Autodesk Fusion 360 part; units mm, degrees
note: some values were not read from the file. Chosen so that the rebuilt part matches the saved one: which bodies a step acts on; which face or edge a step refers to. Set by a fixed rule: which sketch regions a step uses.
(part 2 of 3)
sketch "Sketch1" plane through (0, 0, 0) normal (0, 0, 1) x (1, 0, 0)
  line L0 (10, 10) -> (15, 10)
  line L1 (15, 10) -> (15, 4)
  line L2 (15, 4) -> (10, 4)
  line L3 (10, 4) -> (10, 10)
  line L4 (10, 7) -> (-20, 7) construction
  line L5 (-20, 10) -> (-15, 10)
  line L6 (-15, 10) -> (-15, 4)
  line L7 (-15, 4) -> (-20, 4)
  line L8 (-20, 4) -> (-20, 10)
  dimension "d1" = 5
  dimension "d2" = 6
  dimension "d3" = 30
  dimension "d4" = 5
  dimension "d5" = 6
  constraint horizontal L0
  constraint vertical L1
  constraint horizontal L2
  constraint vertical L3
  constraint midpoint L3 L4.start
  constraint perpendicular L3 L4
  constraint horizontal L5
  constraint vertical L6
  constraint horizontal L7
  constraint vertical L8
  measures "d1" distance of L0.start L0.end
  measures "d2" distance of L0.start L2.end
  measures "d3" distance of L4.start L4.end
  measures "d4" distance of L5.start L5.end
  measures "d5" distance of L5.start L7.end
extrude "Extrude1" add sketch "Sketch1" along normal blind 34.231 makes body 1 at (-15, 8, 11.4103) makes body 2 at (15, 8, 11.4103)
sketch "Sketch2" plane through (-15, 0, 0) normal (1, 0, 0) x (0, 1, 0)
  line L0 (4, 0) -> (10, 0)
  line L1 (10, 0) -> (10, 34.231)
  line L2 (10, 34.231) -> (4, 34.231)
  line L3 (4, 34.231) -> (4, 0)
  line L4 (4, 34.231) -> (10, 34.231)
  line L5 (10, 34.231) -> (10, 29.231)
  line L6 (10, 29.231) -> (4, 29.231)
  line L7 (4, 29.231) -> (4, 34.231)
  dimension "d8" = 5
  constraint horizontal L4
  constraint vertical L5
  constraint horizontal L6
  constraint vertical L7
  constraint coincident L2.end L3.start
  measures "d8" distance of L2.end L6.end
extrude "Extrude2" add sketch "Sketch2" along normal blind 20 contours L1 L2 L3 L4 L5 L6 L7 bodies 1
move_body "Move1" bodies 2 to x (1, 0, 0) y (0, 1, 0) z (0, 0, 1) at (-5, 0, 0)
combine "Combine1" operation add target body 1 tool bodies 2
sketch "Sketch3" plane through (0, 0, 34.231) normal (0, 0, 1) x (-1, 0, 0)
  line L0 (20, -4) -> (-10, -4)
  line L1 (-10, -4) -> (-10, -10)
  line L2 (-10, -10) -> (20, -10)
  line L3 (20, -10) -> (20, -4)
  line L4 (-10, -10) -> (2, -10)
  line L5 (2, -10) -> (2, -4)
  line L6 (2, -4) -> (-10, -4)
  line L7 (-10, -4) -> (-10, -10)
  line L8 (20, -10) -> (8, -10)
  line L9 (8, -10) -> (8, -4)
  line L10 (8, -4) -> (20, -4)
  line L11 (20, -4) -> (20, -10)
  line L12 (2, -10) -> (-3, -10)
  line L13 (-3, -10) -> (-3, -4)
  line L14 (-3, -4) -> (2, -4)
  line L15 (2, -4) -> (2, -10)
  line L16 (8, -10) -> (13, -10)
  line L17 (13, -10) -> (13, -4)
  line L18 (13, -4) -> (8, -4)
  line L19 (8, -4) -> (8, -10)
  constraint horizontal L4
  constraint vertical L5
  constraint horizontal L6
  constraint vertical L7
  constraint coincident L0 L5.end
  constraint coincident L1.end L2.start
  constraint horizontal L8
  constraint vertical L9
  constraint horizontal L10
  constraint vertical L11
  constraint coincident L0 L9.end
  constraint coincident L2.end L3.start
  constraint horizontal L12
  constraint vertical L13
  constraint horizontal L14
  constraint vertical L15
  constraint coincident L6 L13.end
  constraint horizontal L16
  constraint vertical L17
  constraint horizontal L18
  constraint vertical L19
  constraint coincident L10 L17.end
extrude "Extrude3" add sketch "Sketch3" along normal blind 6 contours L0 L2 L8 L9 L10 L16 L17 L18 L19 | L0 L2 L4 L5 L6 L12 L13 L14 L15 bodies 1
extrude "Extrude4" cut 1 faces at (-6, 8, 34.231) along direction (0, 0, -1) blind 5 on bodies 1 bodies 1 makes body 3 at (10, 8, 11.4103)
sketch "Sketch4" plane through (-8, 0, 0) normal (1, 0, 0) x (0, 1, 0)
  line L0 (10, 29.231) -> (10, 40.231)
  line L1 (10, 40.231) -> (4, 40.231)
  line L2 (4, 40.231) -> (4, 29.231)
  line L3 (4, 29.231) -> (10, 29.231)
  line L4 (4, 40.231) -> (10, 40.231)
  line L5 (10, 40.231) -> (10, 34.231)
  line L6 (10, 34.231) -> (4, 34.231)
  line L7 (4, 34.231) -> (4, 40.231)
  dimension "d15" = 6
  constraint horizontal L4
  constraint vertical L5
  constraint horizontal L6
  constraint vertical L7
  constraint coincident L0 L5.end
  constraint coincident L1.end L2.start
  measures "d15" distance of L1.end L6.end
extrude "Extrude5" add sketch "Sketch4" along normal blind 6 contours L0 L1 L2 L4 L5 L6 L7 bodies 1 3
fillet "Fillet1" radius 2 8 edges at (3, 7, 40.231) (3, 7, 34.231) (10, 7, 34.231) (-13, 7, 40.231) (-13, 7, 34.231) (-20, 7, 34.231) (-8, 7, 29.231) (-2, 7, 29.231) on bodies 1
extrude "Extrude6" add 2 faces at (-18.3333, 8, 0) (6.6667, 8, 0) along direction (0, 0, -1) blind 4 on bodies 1 bodies 1
fillet "Fillet2" radius 2 4 edges at (-15, 7, -4) (-20, 7, -4) (5, 7, -4) (10, 7, -4) on bodies 1
sketch "Sketch6" plane through (0, 4, 0) normal (0, -1, 0) x (1, 0, 0)
  arc A0 (8, -4) -> (10, -2) centre (8, -2) ccw
  line L0 (10, -2) -> (10, 32.231)
  arc A1 (10, 32.231) -> (8, 34.231) centre (8, 32.231) ccw
  line L1 (8, 34.231) -> (5, 34.231)
  arc A2 (3, 36.231) -> (5, 34.231) centre (5, 36.231) ccw
  line L2 (3, 36.231) -> (3, 38.231)
  arc A3 (3, 38.231) -> (1, 40.231) centre (1, 38.231) ccw
  line L3 (1, 40.231) -> (-11, 40.231)
  arc A4 (-11, 40.231) -> (-13, 38.231) centre (-11, 38.231) ccw
  line L4 (-13, 38.231) -> (-13, 36.231)
  arc A5 (-15, 34.231) -> (-13, 36.231) centre (-15, 36.231) ccw
  line L5 (-15, 34.231) -> (-18, 34.231)
  arc A6 (-18, 34.231) -> (-20, 32.231) centre (-18, 32.231) ccw
  line L6 (-20, 32.231) -> (-20, -2)
  arc A7 (-20, -2) -> (-18, -4) centre (-18, -2) ccw
  line L7 (-18, -4) -> (-17, -4)
  arc A8 (-17, -4) -> (-15, -2) centre (-17, -2) ccw
  line L8 (-15, -2) -> (-15, 29.231)
  line L9 (-15, 29.231) -> (-10, 29.231)
  arc A9 (-10, 29.231) -> (-8, 31.231) centre (-10, 31.231) ccw
  line L10 (-8, 31.231) -> (-8, 34.231)
  line L11 (-8, 34.231) -> (-2, 34.231)
  line L12 (-2, 34.231) -> (-2, 31.231)
  arc A10 (-2, 31.231) -> (0, 29.231) centre (0, 31.231) ccw
  line L13 (0, 29.231) -> (5, 29.231)
  line L14 (5, 29.231) -> (5, -2)
  arc A11 (5, -2) -> (7, -4) centre (7, -2) ccw
  line L15 (7, -4) -> (8, -4)

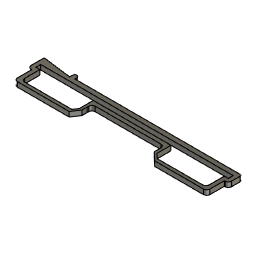
design "Dual Dc and gear"
Autodesk Fusion 360 part; units mm, degrees
sketch "Sketch1" plane through (0, 0, 0) normal (0, 0, 1) x (1, 0, 0)
  line L0 (-83.1348, 11.7496) -> (-83.1348, 16.7496)
  line L1 (-48.4171, -17.3931) -> (-51.4981, -22.0146)
  line L2 (45, -5) -> (45, -17.3931)
  line L3 (-51.4981, -22.0146) -> (-115, -22.0146)
  line L4 (48.3777, -17.3931) -> (48.3777, 0)
  line L5 (55, -27) -> (120, -27)
  line L6 (-115, 0) -> (-120, 0)
  line L7 (-120, 0) -> (-120, 6)
  line L8 (-120, 6) -> (120, 6)
  line L9 (48.3777, 0) -> (-48.4171, 0)
  line L10 (115, -22.0146) -> (53.2559, -22.0146)
  line L11 (53.2559, -22.0146) -> (48.3777, -17.3931)
  line L12 (-88.9, 10.8) -> (-120, 14.8)
  line L13 (125, 11.7496) -> (-83.1348, 11.7496)
  line L14 (-45, -5) -> (45, -5)
  line L15 (-115, -22.0146) -> (-115, 0)
  line L16 (-120, -5) -> (-120, -27.0146)
  line L17 (-48.4171, 0) -> (-48.4171, -17.3931)
  line L18 (-88.1348, 16.7496) -> (-88.9, 10.8)
  line L19 (-45.0838, -17.3931) -> (-45.0838, -11)
  line L20 (-125.0002, -5) -> (-120, -5)
  line L21 (120, -5) -> (125, -5)
  line L22 (120, -27) -> (120, -5)
  line L23 (53.2559, -25.2145) -> (55, -27)
  line L24 (125, -5) -> (125, 11.7496)
  line L25 (-51.4981, -27.0146) -> (-45.0838, -17.3931)
  line L26 (-45.0838, -11) -> (-45, -5)
  line L27 (-120, -27.0146) -> (-51.4981, -27.0146)
  line L28 (-125.0002, 15.4377) -> (-125.0002, -5)
  line L29 (115, 0) -> (115, -22.0146)
  line L30 (-83.1348, 16.7496) -> (-88.1348, 16.7496)
  line L31 (120, 6) -> (120, 0)
  line L32 (-120, 14.8) -> (-125.0002, 15.4377)
  line L33 (45, -17.3931) -> (53.2559, -25.2145)
  line L34 (120, 0) -> (115, 0)
extrude "Extrude1" add sketch "Sketch1" along normal blind 6
fillet "Fillet1" radius 4 6 edges at (120, -27, 3) (125, -5, 3) (45, -5, 3) (-45, -5, 3) (-120, -27.0146, 3) (-125.0002, -5, 3)
sketch "Sketch2" plane through (0, 0, 6) normal (0, 0, 1) x (-1, 0, 0)
  arc A0 (125.0002, 1) -> (121.0002, 5) centre (121.0002, 1) ccw
  line L0 (121.0002, 5) -> (120, 5)
  line L1 (120, 5) -> (120, 23.0146)
  arc A1 (120, 23.0146) -> (116, 27.0146) centre (116, 23.0146) ccw
  line L2 (116, 27.0146) -> (51.4981, 27.0146)
  line L3 (51.4981, 27.0146) -> (45.0838, 17.3931)
  line L4 (45.0838, 17.3931) -> (45.0838, 11)
  line L5 (45.0838, 11) -> (45.0551, 8.9442)
  arc A2 (41.0555, 5) -> (45.0551, 8.9442) centre (41.0555, 9) ccw
  line L6 (41.0555, 5) -> (-41, 5)
  arc A3 (-45, 9) -> (-41, 5) centre (-41, 9) ccw
  line L7 (-45, 9) -> (-45, 17.3931)
  line L8 (-45, 17.3931) -> (-53.2559, 25.2145)
  line L9 (-53.2559, 25.2145) -> (-55, 27)
  line L10 (-55, 27) -> (-116, 27)
  arc A4 (-116, 27) -> (-120, 23) centre (-116, 23) ccw
  line L11 (-120, 23) -> (-120, 5)
  line L12 (-120, 5) -> (-121, 5)
  arc A5 (-121, 5) -> (-125, 1) centre (-121, 1) ccw
  line L13 (-125, 1) -> (-125, -11.7496)
  line L14 (-125, -11.7496) -> (83.1348, -11.7496)
  line L15 (83.1348, -11.7496) -> (83.1348, -16.7496)
  line L16 (83.1348, -16.7496) -> (88.1348, -16.7496)
  line L17 (88.1348, -16.7496) -> (88.9, -10.8)
  line L18 (88.9, -10.8) -> (120, -14.8)
  line L19 (120, -14.8) -> (125.0002, -15.4377)
  line L20 (125.0002, -15.4377) -> (125.0002, 1)
  line L21 (-120, -6) -> (-120, 0)
  line L22 (-120, 0) -> (-115, 0)
  line L23 (-115, 0) -> (-115, 22.0146)
  line L24 (-115, 22.0146) -> (-53.2559, 22.0146)
  line L25 (-53.2559, 22.0146) -> (-48.3777, 17.3931)
  line L26 (-48.3777, 17.3931) -> (-48.3777, 0)
  line L27 (-48.3777, 0) -> (48.4171, 0)
  line L28 (48.4171, 0) -> (48.4171, 17.3931)
  line L29 (48.4171, 17.3931) -> (51.4981, 22.0146)
  line L30 (51.4981, 22.0146) -> (115, 22.0146)
  line L31 (115, 22.0146) -> (115, 0)
  line L32 (115, 0) -> (120, 0)
  line L33 (120, 0) -> (120, -6)
  line L34 (120, -6) -> (-120, -6)
  line L35 (-115, 22.0146) -> (-115, 23.0146)
  line L36 (-115, 23.0146) -> (-54.3115, 23.0146)
  line L37 (-54.3115, 23.0146) -> (-53.2559, 22.0146)
  dimension "d7" = 1
  constraint coincident L23.end L24.start
  constraint perpendicular L24 L35
  constraint perpendicular L35 L36
  constraint coincident L24.end L25.start
  constraint parallel L25 L37
  measures "d7" distance of L23.end L35.end
extrude "Extrude2" cut sketch "Sketch2" against normal blind 14 contours L24 L35 L36 L37
fillet "Fillet3" radius 4 1 edges at (115, -23.0146, 3)
sketch "Sketch3" plane through (0, 0, 6) normal (0, 0, 1) x (-1, 0, 0)
  line L0 (-115, 0) -> (-115, 19.0146)
  arc A0 (-111, 23.0146) -> (-115, 19.0146) centre (-111, 19.0146) ccw
  line L1 (-111, 23.0146) -> (-54.3115, 23.0146)
  line L2 (-54.3115, 23.0146) -> (-48.3777, 17.3931)
  line L3 (-48.3777, 17.3931) -> (-48.3777, 0)
  line L4 (-48.3777, 0) -> (48.4171, 0)
  line L5 (48.4171, 0) -> (48.4171, 17.3931)
  line L6 (48.4171, 17.3931) -> (51.4981, 22.0146)
  line L7 (51.4981, 22.0146) -> (115, 22.0146)
  line L8 (115, 22.0146) -> (115, 0)
  line L9 (115, 0) -> (120, 0)
  line L10 (120, 0) -> (120, -6)
  line L11 (120, -6) -> (-120, -6)
  line L12 (-120, -6) -> (-120, 0)
  line L13 (-120, 0) -> (-115, 0)
  arc A1 (125.0002, 1) -> (121.0002, 5) centre (121.0002, 1) ccw
  line L14 (121.0002, 5) -> (120, 5)
  line L15 (120, 5) -> (120, 23.0146)
  arc A2 (120, 23.0146) -> (116, 27.0146) centre (116, 23.0146) ccw
  line L16 (116, 27.0146) -> (51.4981, 27.0146)
  line L17 (51.4981, 27.0146) -> (45.0838, 17.3931)
  line L18 (45.0838, 17.3931) -> (45.0838, 11)
  line L19 (45.0838, 11) -> (45.0551, 8.9442)
  arc A3 (41.0555, 5) -> (45.0551, 8.9442) centre (41.0555, 9) ccw
  line L20 (41.0555, 5) -> (-41, 5)
  arc A4 (-45, 9) -> (-41, 5) centre (-41, 9) ccw
  line L21 (-45, 9) -> (-45, 17.3931)
  line L22 (-45, 17.3931) -> (-53.2559, 25.2145)
  line L23 (-53.2559, 25.2145) -> (-55, 27)
  line L24 (-55, 27) -> (-116, 27)
  arc A5 (-116, 27) -> (-120, 23) centre (-116, 23) ccw
  line L25 (-120, 23) -> (-120, 5)
  line L26 (-120, 5) -> (-121, 5)
  arc A6 (-121, 5) -> (-125, 1) centre (-121, 1) ccw
  line L27 (-125, 1) -> (-125, -11.7496)
  line L28 (-125, -11.7496) -> (83.1348, -11.7496)
  line L29 (83.1348, -11.7496) -> (83.1348, -16.7496)
  line L30 (83.1348, -16.7496) -> (88.1348, -16.7496)
  line L31 (88.1348, -16.7496) -> (88.9, -10.8)
  line L32 (88.9, -10.8) -> (120, -14.8)
  line L33 (120, -14.8) -> (125.0002, -15.4377)
  line L34 (125.0002, -15.4377) -> (125.0002, 1)
  line L35 (115, 22.0146) -> (115, 23.0146)
  line L36 (115, 23.0146) -> (52.1648, 23.0146)
  line L37 (52.1648, 23.0146) -> (51.4981, 22.0146)
  dimension "d12" = 1
  constraint coincident L7.end L8.start
  constraint perpendicular L7 L35
  constraint perpendicular L8 L36
  constraint coincident L6.end L7.start
  constraint parallel L6 L37
  measures "d12" distance of L7.end L35.end
extrude "Extrude3" cut sketch "Sketch3" against normal blind 12 contours L7 L35 L36 L37
fillet "Fillet4" radius 4 1 edges at (-115, -23.0146, 3)
fillet "Fillet5" radius 2 1 edges at (125, 11.7496, 3)
fillet "Fillet6" radius 2 1 edges at (-83.1348, 16.7496, 3)
fillet "Fillet7" radius 1 1 edges at (115, 0, 3)
sketch "Sketch4" plane through (0, 0, 6) normal (0, 0, 1) x (-1, 0, 0)
  arc A0 (-116, 0) -> (-115, 1) centre (-116, 1) ccw
  line L0 (-115, 1) -> (-115, 19.0146)
  arc A1 (-111, 23.0146) -> (-115, 19.0146) centre (-111, 19.0146) ccw
  line L1 (-111, 23.0146) -> (-54.3115, 23.0146)
  line L2 (-54.3115, 23.0146) -> (-48.3777, 17.3931)
  line L3 (-48.3777, 17.3931) -> (-48.3777, 0)
  line L4 (-48.3777, 0) -> (48.4171, 0)
  line L5 (48.4171, 0) -> (48.4171, 17.3931)
  line L6 (48.4171, 17.3931) -> (52.1648, 23.0146)
  line L7 (52.1648, 23.0146) -> (111, 23.0146)
  arc A2 (115, 19.0146) -> (111, 23.0146) centre (111, 19.0146) ccw
  line L8 (115, 19.0146) -> (115, 0)
  line L9 (115, 0) -> (120, 0)
  line L10 (120, 0) -> (120, -6)
  line L11 (120, -6) -> (-120, -6)
  line L12 (-120, -6) -> (-120, 0)
  line L13 (-120, 0) -> (-116, 0)
  arc A3 (83.1348, -14.7496) -> (85.1348, -16.7496) centre (85.1348, -14.7496) ccw
  line L14 (85.1348, -16.7496) -> (88.1348, -16.7496)
  line L15 (88.1348, -16.7496) -> (88.9, -10.8)
  line L16 (88.9, -10.8) -> (120, -14.8)
  line L17 (120, -14.8) -> (125.0002, -15.4377)
  line L18 (125.0002, -15.4377) -> (125.0002, 1)
  arc A4 (125.0002, 1) -> (121.0002, 5) centre (121.0002, 1) ccw
  line L19 (121.0002, 5) -> (120, 5)
  line L20 (120, 5) -> (120, 23.0146)
  arc A5 (120, 23.0146) -> (116, 27.0146) centre (116, 23.0146) ccw
  line L21 (116, 27.0146) -> (51.4981, 27.0146)
  line L22 (51.4981, 27.0146) -> (45.0838, 17.3931)
  line L23 (45.0838, 17.3931) -> (45.0838, 11)
  line L24 (45.0838, 11) -> (45.0551, 8.9442)
  arc A6 (41.0555, 5) -> (45.0551, 8.9442) centre (41.0555, 9) ccw
  line L25 (41.0555, 5) -> (-41, 5)
  arc A7 (-45, 9) -> (-41, 5) centre (-41, 9) ccw
  line L26 (-45, 9) -> (-45, 17.3931)
  line L27 (-45, 17.3931) -> (-53.2559, 25.2145)
  line L28 (-53.2559, 25.2145) -> (-55, 27)
  line L29 (-55, 27) -> (-116, 27)
  arc A8 (-116, 27) -> (-120, 23) centre (-116, 23) ccw
  line L30 (-120, 23) -> (-120, 5)
  line L31 (-120, 5) -> (-121, 5)
  arc A9 (-121, 5) -> (-125, 1) centre (-121, 1) ccw
  line L32 (-125, 1) -> (-125, -9.7496)
  arc A10 (-125, -9.7496) -> (-123, -11.7496) centre (-123, -9.7496) ccw
  line L33 (-123, -11.7496) -> (83.1348, -11.7496)
  line L34 (83.1348, -11.7496) -> (83.1348, -14.7496)

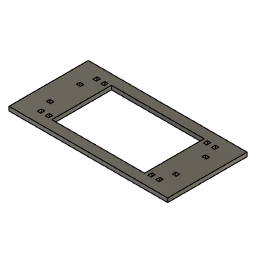
design "Test Base"
Autodesk Fusion 360 part; units mm, degrees
sketch "Sketch1" plane through (0, 0, 0) normal (0, 0, 1) x (1, 0, 0) in component "Base"
  line L0 (120, 60) -> (-120, 60)
  line L1 (-120, 60) -> (-120, -60)
  line L2 (-120, -60) -> (120, -60)
  line L3 (120, -60) -> (120, 60)
  line L4 (120, 60) -> (-120, -60) construction
  line L5 (-120, 60) -> (120, -60) construction
  line L6 (-70, 45) -> (70, 45)
  line L7 (70, 45) -> (70, -45)
  line L8 (70, -45) -> (-70, -45)
  line L9 (-70, -45) -> (-70, 45)
  line L10 (-70, 45) -> (70, -45) construction
  line L11 (70, 45) -> (-70, -45) construction
  dimension "d1" = 240
  dimension "d2" = 120
  dimension "d3" = 90
  dimension "d6" = 140
  constraint horizontal L0
  constraint perpendicular L0 L1
  constraint parallel L0 L2
  constraint parallel L1 L3
  constraint coincident L4 origin
  constraint coincident L5 origin
  constraint horizontal L6
  constraint perpendicular L6 L7
  constraint parallel L6 L8
  constraint parallel L7 L9
  constraint coincident L10 origin
  constraint coincident L11 origin
  measures "d1" distance of L1.end L2.end
  measures "d2" distance of L0.end L1.end
  measures "d3" distance of L6.end L7.end
  measures "d6" distance of L7 L9
extrude "Extrude1" add sketch "Sketch1" along normal blind 6 in component "Base"
sketch "Sketch2" plane through (0, 0, 6) normal (0, 0, 1) x (-1, 0, 0) in component "Base"
  line L0 (-70, 45) -> (70, 45)
  line L1 (70, 45) -> (70, -45)
  line L2 (70, -45) -> (-70, -45)
  line L3 (-70, -45) -> (-70, 45)
  line L4 (-120, 60) -> (-120, -60)
  line L5 (-120, -60) -> (120, -60)
  line L6 (120, -60) -> (120, 60)
  line L7 (120, 60) -> (-120, 60)
  line L8 (70, 45) -> (92, 45) construction
  line L9 (92, 45) -> (92, 39) construction
  line L10 (92, 39) -> (70, 39) construction
  line L11 (70, 39) -> (70, 45) construction
  line L12 (92, 39) -> (87, 39)
  line L13 (87, 39) -> (87, 45)
  line L14 (87, 45) -> (92, 45)
  line L15 (92, 45) -> (92, 39)
  line L16 (70, 39) -> (75, 39) construction
  line L17 (75, 45) -> (75, 39) construction
  line L18 (75, 39) -> (80, 39)
  line L19 (80, 39) -> (80, 45)
  line L20 (80, 45) -> (75, 45)
  line L21 (75, 45) -> (75, 39)
  dimension "d15" = 6
  constraint horizontal L8
  constraint vertical L9
  constraint horizontal L10
  constraint vertical L11
  constraint coincident L0.end L1.start
  constraint horizontal L12
  constraint vertical L13
  constraint horizontal L14
  constraint vertical L15
  constraint coincident L8 L13.end
  constraint coincident L10 L16.end
  constraint coincident L8 L17.start
  constraint perpendicular L10 L17
  constraint horizontal L18
  constraint vertical L19
  constraint horizontal L20
  constraint vertical L21
  constraint coincident L8 L19.end
  measures "d15" distance of L8 L12
extrude "Extrude2" cut sketch "Sketch2" against normal blind 6 contours L12 L13 L14 L15 | L18 L19 L20 L21 in component "Base"
ref_plane "WorkPlane1" through (0, 0, 0) normal (1, 0, 0) x (0, 1, 0) in component "Base"
mirror "Mirror1" about plane through (0, 0, 0) normal (1, 0, 0) of "Extrude2" in component "Base"
ref_plane "WorkPlane2" through (0, 0, 0) normal (0, 1, 0) x (0, 0, 1) in component "Base"
mirror "Mirror2" about plane through (0, 0, 0) normal (0, 1, 0) of "Extrude2", "Mirror1" in component "Base"
sketch "Sketch3" plane through (0, 0, 0) normal (0, 0, -1) x (1, 0, 0) in component "Base"
  line L0 (87, -45) -> (87, -39)
  line L1 (87, -39) -> (92, -39)
  line L2 (92, -39) -> (92, -45)
  line L3 (92, -45) -> (87, -45)
  line L4 (75, -39) -> (80, -39)
  line L5 (80, -39) -> (80, -45)
  line L6 (80, -45) -> (75, -45)
  line L7 (75, -45) -> (75, -39)
  line L8 (-87, -39) -> (-87, -45)
  line L9 (-87, -45) -> (-92, -45)
  line L10 (-92, -45) -> (-92, -39)
  line L11 (-92, -39) -> (-87, -39)
  line L12 (-80, -39) -> (-75, -39)
  line L13 (-75, -39) -> (-75, -45)
  line L14 (-75, -45) -> (-80, -45)
  line L15 (-80, -45) -> (-80, -39)
  line L16 (87, 39) -> (87, 45)
  line L17 (87, 45) -> (92, 45)
  line L18 (92, 45) -> (92, 39)
  line L19 (92, 39) -> (87, 39)
  line L20 (80, 39) -> (75, 39)
  line L21 (75, 39) -> (75, 45)
  line L22 (75, 45) -> (80, 45)
  line L23 (80, 45) -> (80, 39)
  line L24 (-87, 45) -> (-87, 39)
  line L25 (-87, 39) -> (-92, 39)
  line L26 (-92, 39) -> (-92, 45)
  line L27 (-92, 45) -> (-87, 45)
  line L28 (-75, 39) -> (-80, 39)
  line L29 (-80, 39) -> (-80, 45)
  line L30 (-80, 45) -> (-75, 45)
  line L31 (-75, 45) -> (-75, 39)
  line L32 (-70, 45) -> (70, 45)
  line L33 (70, 45) -> (70, -45)
  line L34 (70, -45) -> (-70, -45)
  line L35 (-70, -45) -> (-70, 45)
  line L36 (120, -60) -> (120, 60)
  line L37 (120, 60) -> (-120, 60)
  line L38 (-120, 60) -> (-120, -60)
  line L39 (-120, -60) -> (120, -60)
  line L40 (-120, 0) -> (-70, 0) construction
  line L41 (-87, -39) -> (-87, 39) construction
  line L42 (-87, 0) -> (-87, -20) construction
  line L43 (-87, 0) -> (-87, -20) construction
  line L44 (-87, 0) -> (-93, 0) construction
  line L45 (-87, 0) -> (-92, 0) construction
  line L46 (-92, 0) -> (-92, -20) construction
  line L47 (-92, -20) -> (-87, -20) construction
  line L48 (-87, -20) -> (-87, 0) construction
  line L49 (-87, 0) -> (-91.9449, 0) construction
  line L50 (-91.9449, 20) -> (-87, 20) construction
  line L51 (-87, 20) -> (-87, 0) construction
  line L52 (-87, 0) -> (-92, 0) construction
  line L53 (-92, 0) -> (-92, 20) construction
  line L54 (-92, 20) -> (-87, 20) construction
  line L55 (-87, 20) -> (-87, 0) construction
  line L56 (-92, -20) -> (-98, -20)
  line L57 (-98, -20) -> (-98, -25)
  line L58 (-98, -25) -> (-92, -25)
  line L59 (-92, -25) -> (-92, -20)
  line L60 (-92, 20) -> (-98, 20)
  line L61 (-98, 20) -> (-98, 25)
  line L62 (-98, 25) -> (-92, 25)
  line L63 (-92, 25) -> (-92, 20)
  dimension "d16" = 5
  dimension "d17" = 20
  dimension "d18" = 20
  constraint midpoint L38 L40.start
  constraint midpoint L35 L40.end
  constraint coincident L8.start L11.end
  constraint coincident L24.end L25.start
  constraint midpoint L41 L42.start
  constraint coincident L41 L42.end
  constraint perpendicular L40 L42
  constraint coincident L40 L44.end
  constraint perpendicular L41 L44
  constraint horizontal L45
  constraint vertical L46
  constraint horizontal L47
  constraint vertical L48
  constraint horizontal L49
  constraint horizontal L50
  constraint vertical L51
  constraint horizontal L52
  constraint vertical L53
  constraint horizontal L54
  constraint vertical L55
  constraint horizontal L56
  constraint vertical L57
  constraint horizontal L58
  constraint vertical L59
  constraint horizontal L60
  constraint vertical L61
  constraint horizontal L62
  constraint vertical L63
  measures "d16" distance of L42.start L45.end
  measures "d17" distance of L42.start L42.end
  measures "d18" distance of L42.start L50.end
extrude "Extrude3" cut sketch "Sketch3" against normal blind 11 contours L56 L57 L58 L59 | L60 L61 L62 L63 in component "Base"
mirror "Mirror3" about plane through (0, 0, 0) normal (1, 0, 0) of "Extrude3" in component "Base"
component "Base" placed x (1, 0, 0) y (0, 1, 0) z (0, 0, 1) at (0, 0, 0)

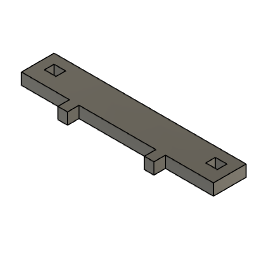
design "North/South Plank"
Autodesk Fusion 360 part; units mm, degrees
sketch "Sketch1" plane through (0, 0, 0) normal (0, 0, 1) x (1, 0, 0)
  line L0 (-45, 8.5) -> (45, 8.5)
  line L1 (45, 8.5) -> (45, -8.5)
  line L2 (45, -8.5) -> (-45, -8.5)
  line L3 (-45, -8.5) -> (-45, 8.5)
  line L4 (-45, 8.5) -> (45, -8.5) construction
  line L5 (45, 8.5) -> (-45, -8.5) construction
  dimension "d1" = 90
  dimension "d2" = 17
  constraint horizontal L0
  constraint perpendicular L0 L1
  constraint parallel L0 L2
  constraint parallel L1 L3
  constraint coincident L4 origin
  constraint coincident L5 origin
  measures "d1" distance of L1.end L2.end
  measures "d2" distance of L0.end L1.end
extrude "Extrude1" add sketch "Sketch1" along normal blind 6
sketch "Sketch2" plane through (0, 0, 6) normal (0, 0, 1) x (-1, 0, 0)
  line L0 (45, 8.5) -> (-45, 8.5)
  line L1 (-45, 8.5) -> (-45, -8.5)
  line L2 (-45, -8.5) -> (45, -8.5)
  line L3 (45, -8.5) -> (45, 8.5)
  line L4 (45, -8.5) -> (39, -8.5) construction
  line L5 (39, -8.5) -> (39, -3.5) construction
  line L6 (39, -3.5) -> (45, -3.5) construction
  line L7 (45, -3.5) -> (45, -8.5) construction
  line L8 (-45, -8.5) -> (-39, -8.5) construction
  line L9 (-39, -8.5) -> (-39, -3.5) construction
  line L10 (-39, -3.5) -> (-45, -3.5) construction
  line L11 (-45, -3.5) -> (-45, -8.5) construction
  line L12 (45, -3.5) -> (39, -3.5)
  line L13 (39, -3.5) -> (39, 1.5)
  line L14 (39, 1.5) -> (45, 1.5)
  line L15 (45, 1.5) -> (45, -3.5)
  line L16 (-45, -3.5) -> (-39, -3.5)
  line L17 (-39, -3.5) -> (-39, 1.5)
  line L18 (-39, 1.5) -> (-45, 1.5)
  line L19 (-45, 1.5) -> (-45, -3.5)
  dimension "d5" = 6
  dimension "d6" = 5
  dimension "d7" = 6
  dimension "d8" = 5
  dimension "d9" = 5
  dimension "d10" = 5
  constraint horizontal L4
  constraint vertical L5
  constraint horizontal L6
  constraint vertical L7
  constraint coincident L2.end L3.start
  constraint horizontal L8
  constraint vertical L9
  constraint horizontal L10
  constraint vertical L11
  constraint coincident L1.end L2.start
  constraint horizontal L12
  constraint vertical L13
  constraint horizontal L14
  constraint vertical L15
  constraint horizontal L16
  constraint vertical L17
  constraint horizontal L18
  constraint vertical L19
  measures "d5" distance of L2.end L4.end
  measures "d6" distance of L2.end L6.end
  measures "d7" distance of L1.end L8.end
  measures "d8" distance of L1.end L10.end
  measures "d9" distance of L6.end L14.end
  measures "d10" distance of L10.end L18.end
extrude "Extrude2" cut sketch "Sketch2" against normal blind 9 contours L3 L12 L13 L14 L15 | L1 L16 L17 L18 L19
sketch "Sketch3" plane through (0, -8.5, 0) normal (0, -1, 0) x (1, 0, 0)
  line L0 (-45, 0) -> (45, 0)
  line L1 (45, 0) -> (45, 6)
  line L2 (45, 6) -> (-45, 6)
  line L3 (-45, 6) -> (-45, 0)
  line L4 (0, 6) -> (39, 6) construction
  line L5 (39, 0) -> (39, 6) construction
  line L6 (0, 6) -> (-39, 6) construction
  line L7 (-39, 6) -> (-39, 0) construction
  line L8 (0, 6) -> (0, 0)
  line L9 (0, 2.5249) -> (-20, 2.5249) construction
  line L10 (-20, 2.5249) -> (-20, 0) construction
  line L11 (0, 2.5249) -> (20, 2.5249) construction
  line L12 (-20, 0) -> (-25, 0)
  line L13 (-25, 0) -> (-25, 6)
  line L14 (-25, 6) -> (-20, 6)
  line L15 (-20, 6) -> (-20, 0)
  line L16 (20, 0) -> (25, 0)
  line L17 (25, 0) -> (25, 6)
  line L18 (25, 6) -> (20, 6)
  line L19 (20, 6) -> (20, 0)
  constraint midpoint L2 L4.start
  constraint coincident L2 L4.end
  constraint parallel L2 L4
  constraint coincident L0 L5.start
  constraint perpendicular L4 L5
  constraint coincident L2 L6.end
  constraint perpendicular L5 L6
  constraint coincident L0 L7.end
  constraint perpendicular L0 L7
  constraint coincident L8.end origin
  constraint coincident L8 L9.start
  constraint perpendicular L8 L9
  constraint coincident L0 L10.end
  constraint perpendicular L0 L10
  constraint perpendicular L8 L11
  constraint horizontal L12
  constraint vertical L13
  constraint horizontal L14
  constraint vertical L15
  constraint coincident L6 L13.end
  constraint horizontal L16
  constraint vertical L17
  constraint horizontal L18
  constraint vertical L19
  constraint coincident L4 L17.end
  constraint coincident L0 L16.start
extrude "Extrude3" add sketch "Sketch3" along normal blind 6 contours L0 L2 L12 L13 L14 L15 | L0 L2 L16 L17 L18 L19
sketch "Sketch4" plane through (-45, 0, 0) normal (-1, 0, 0) x (0, -1, 0)
  line L0 (-3.5, 0) -> (-3.5, 6)
  line L1 (-3.5, 6) -> (-8.5, 6)
  line L2 (-8.5, 6) -> (-8.5, 0)
  line L3 (-8.5, 0) -> (-3.5, 0)
  line L4 (-8.5, 6) -> (8.5, 6)
  line L5 (8.5, 6) -> (8.5, 0)
  line L6 (8.5, 0) -> (-8.5, 0)
  line L7 (-8.5, 0) -> (-8.5, 6)
  dimension "d15" = 17
  dimension "d16" = 6
  constraint horizontal L4
  constraint vertical L5
  constraint horizontal L6
  constraint vertical L7
  constraint coincident L1.end L2.start
  measures "d15" distance of L1.end L4.end
  measures "d16" distance of L1.end L2.end
extrude "Extrude4" add sketch "Sketch4" along normal blind 5
sketch "Sketch5" plane through (45, 0, 0) normal (1, 0, 0) x (0, 1, 0)
  line L0 (-1.5, 0) -> (-1.5, 6)
  line L1 (-1.5, 6) -> (-8.5, 6)
  line L2 (-8.5, 6) -> (-8.5, 0)
  line L3 (-8.5, 0) -> (-1.5, 0)
  line L4 (-8.5, 6) -> (8.5, 6)
  line L5 (8.5, 6) -> (8.5, 0)
  line L6 (8.5, 0) -> (-8.5, 0)
  line L7 (-8.5, 0) -> (-8.5, 6)
  dimension "d19" = 17
  constraint horizontal L4
  constraint vertical L5
  constraint horizontal L6
  constraint vertical L7
  constraint coincident L1.end L2.start
  measures "d19" distance of L1.end L4.end
extrude "Extrude5" add sketch "Sketch5" along normal blind 5

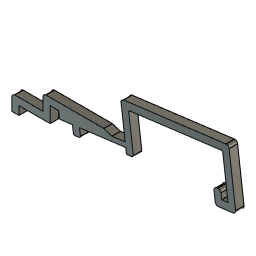
design "HOOK ARM"
Autodesk Fusion 360 part; units mm, degrees
ref_plane "WorkPlane1" through (112.1576, 66, 17) normal (0, 1, 0) x (-1, 0, 0)
sketch "Sketch2" plane through (0, 66, 0) normal (0, 1, 0) x (1, 0, 0)
  line L0 (87, -6) -> (87, -28)
  line L1 (87, -28) -> (130, -28)
  line L2 (130, -28) -> (136, -26)
  line L3 (136, -26) -> (137, -23)
  line L4 (137, -23) -> (98, -18)
  line L5 (98, -18) -> (98, -23)
  line L6 (98, -23) -> (92, -23)
  line L7 (92, -23) -> (92, -6)
  line L8 (92, -6) -> (87, -6)
  constraint vertical L0
  constraint perpendicular L0 L1
  constraint perpendicular L1 L5
  constraint perpendicular L5 L6
  constraint perpendicular L6 L7
  constraint perpendicular L7 L8
extrude "Extrude1" add sketch "Sketch2" along normal blind 6 makes body 1
sketch "Sketch3" plane through (-0.6856, 0, 5.348) normal (0.127164, 0, -0.991882) x (0, 1, 0)
  line L0 (66, 138.8126) -> (66, 99.4934)
  line L1 (66, 99.4934) -> (72, 99.4934)
  line L2 (72, 99.4934) -> (72, 138.8126)
  line L3 (72, 138.8126) -> (66, 138.8126)
  line L4 (69.556, 99.4934) -> (69.556, 104.3824) construction
  line L5 (72, 104.3824) -> (66, 104.3824)
  line L6 (66, 104.3824) -> (66, 109.3824)
  line L7 (66, 109.3824) -> (72, 109.3824)
  line L8 (72, 109.3824) -> (72, 104.3824)
  line L9 (72, 109.3824) -> (66, 109.3824)
  line L10 (66, 109.3824) -> (66, 114.3824)
  line L11 (66, 114.3824) -> (72, 114.3824)
  line L12 (72, 114.3824) -> (72, 109.3824)
  dimension "d4" = 4.889
  dimension "d5" = 5
  dimension "d46" = 5
  constraint coincident L1 L4.start
  constraint perpendicular L1 L4
  constraint horizontal L5
  constraint vertical L6
  constraint horizontal L7
  constraint vertical L8
  constraint coincident L2 L5.start
  constraint horizontal L9
  constraint vertical L10
  constraint horizontal L11
  constraint vertical L12
  constraint coincident L0 L10.end
  measures "d4" distance of L4.start L4.end
  measures "d5" distance of L5.start L7.end
  measures "d46" distance of L7.end L11.end
sketch "Sketch4" plane through (0, 72, 0) normal (0, 1, 0) x (-1, 0, 0)
  line L0 (-137, 23) -> (-98, 18)
  line L1 (-98, 18) -> (-98, 23)
  line L2 (-98, 23) -> (-92, 23)
  line L3 (-92, 23) -> (-92, 6)
  line L4 (-92, 6) -> (-87, 6)
  line L5 (-87, 6) -> (-87, 28)
  line L6 (-87, 28) -> (-130, 28)
  line L7 (-130, 28) -> (-136, 26)
  line L8 (-136, 26) -> (-137, 23)
  line L9 (-87, 6) -> (-92, 6)
  line L10 (-92, 6) -> (-92, 12)
  line L11 (-92, 12) -> (-87, 12)
  line L12 (-87, 12) -> (-87, 6)
  line L13 (-87, 12) -> (-65, 12)
  line L14 (-65, 6) -> (-65, 12)
  line L15 (-65, 17) -> (-87, 17)
  line L16 (-65, 6) -> (-70, 6)
  line L17 (-70, 6) -> (-70, 12)
  line L18 (-70, 12) -> (-65, 12)
  line L19 (-65, 12) -> (-65, 6)
  line L20 (-65, 12) -> (-65, 17)
  constraint horizontal L9
  constraint vertical L10
  constraint horizontal L11
  constraint vertical L12
  constraint coincident L3 L10.end
  constraint coincident L4.end L5.start
  constraint perpendicular L5 L13
  constraint perpendicular L13 L14
  constraint midpoint L5 L15.end
  constraint perpendicular L5 L15
  constraint horizontal L16
  constraint vertical L17
  constraint horizontal L18
  constraint vertical L19
  constraint coincident L13 L17.end
  constraint perpendicular L18 L20
extrude "Extrude3" cut sketch "Sketch4" against normal blind 6.5 contours L3 L4 L5 L9 L10 L11 L12 bodies 1
extrude "Extrude4" add sketch "Sketch4" against normal blind 6 contours L5 L13 L15 L18 L20 | L13 L14 L16 L17 L18 L19 bodies 1
sketch "Sketch5" plane through (-0.6856, 0, 5.348) normal (0.127164, 0, -0.991882) x (0, 1, 0)
  line L0 (72, 99.4934) -> (72, 138.8126)
  line L1 (72, 138.8126) -> (66, 138.8126)
  line L2 (66, 138.8126) -> (66, 99.4934)
  line L3 (69, 109.3824) -> (69, 147.2714) construction
  line L4 (69, 147.2714) -> (66, 147.2714) construction
  line L5 (66, 147.2714) -> (66, 144.7714) construction
  line L6 (66, 144.7714) -> (69, 144.7714) construction
  line L7 (69, 144.7714) -> (69, 147.2714) construction
  line L8 (66, 144.7714) -> (72, 144.7714)
  line L9 (72, 144.7714) -> (72, 149.7714)
  line L10 (72, 149.7714) -> (66, 149.7714)
  line L11 (66, 149.7714) -> (66, 144.7714)
  line L12 (66, 99.4934) -> (72, 99.4934)
  dimension "d21" = 37.889
  dimension "d22" = 2.5
  dimension "d23" = 5
  constraint perpendicular L1 L3
  constraint horizontal L4
  constraint vertical L5
  constraint horizontal L6
  constraint vertical L7
  constraint horizontal L8
  constraint vertical L9
  constraint horizontal L10
  constraint vertical L11
  measures "d21" distance of L3.start L3.end
  measures "d22" distance of L3.end L6.end
  measures "d23" distance of L5.end L10.end
sketch "Sketch6" plane through (0, 66, 0) normal (0, -1, 0) x (1, 0, 0)
  line L0 (65, 17) -> (65, 6)
  line L1 (70, 12) -> (92, 12)
  line L2 (92, 12) -> (92, 23)
  line L3 (92, 23) -> (98, 23)
  line L4 (98, 23) -> (98, 18)
  line L5 (98, 18) -> (137, 23)
  line L6 (137, 23) -> (136, 26)
  line L7 (136, 26) -> (130, 28)
  line L8 (130, 28) -> (87, 28)
  line L9 (87, 28) -> (87, 17)
  line L10 (87, 17) -> (65, 17)
  line L11 (136.0676, 22.8805) -> (135.6529, 26.1157)
  line L12 (65, 6) -> (70, 6)
  line L13 (70, 6) -> (70, 12)
  constraint coincident L5 L11.start
  constraint coincident L7 L11.end
  constraint perpendicular L5 L11
extrude "Extrude5" cut sketch "Sketch6" against normal blind 6.8 contours L5 L6 L7 L11 bodies 1
extrude "Extrude6" add 1 faces at (135.9294, 68, 23.9589) along direction (0.991882, 0, 0.127164) blind 14.461 on bodies 1 bodies 1
sketch "Sketch7" plane through (-1.1004, 0, 8.5832) normal (-0.127164, 0, 0.991882) x (0, -1, 0)
  line L0 (-72, 137.8726) -> (-66, 137.8726)
  line L1 (-66, 137.8726) -> (-66, 152.3336)
  line L2 (-66, 152.3336) -> (-72, 152.3336)
  line L3 (-72, 152.3336) -> (-72, 137.8726)
  line L4 (-66, 152.3336) -> (-72.8279, 152.3336)
  line L5 (-72.8279, 152.3336) -> (-72.8279, 147.3336)
  line L6 (-72.8279, 147.3336) -> (-66, 147.3336)
  line L7 (-66, 147.3336) -> (-66, 152.3336)
  dimension "d30" = 5
  constraint horizontal L4
  constraint vertical L5
  constraint horizontal L6
  constraint vertical L7
  constraint coincident L1.end L2.start
  measures "d30" distance of L1.end L6.end
extrude "Extrude8" add sketch "Sketch7" along normal blind 30 contours L1 L2 L3 L4 L6 L7 bodies 1
sketch "Sketch8" plane through (151.0969, 0, 19.3714) normal (0.991882, 0, 0.127164) x (0, 1, 0)
  line L0 (72, 5.3918) -> (72, 38.6535)
  line L1 (72, 38.6535) -> (66, 38.6535)
  line L2 (66, 38.6535) -> (66, 5.3918)
  line L3 (66, 38.6535) -> (72, 38.6535)
  line L4 (72, 38.6535) -> (72, 33.6535)
  line L5 (72, 33.6535) -> (66, 33.6535)
  line L6 (66, 33.6535) -> (66, 38.6535)
  line L7 (66, 5.3918) -> (72, 5.3918)
  dimension "d33" = 5
  constraint horizontal L3
  constraint vertical L4
  constraint horizontal L5
  constraint vertical L6
  constraint coincident L1.end L2.start
  measures "d33" distance of L1.end L5.end
extrude "Extrude9" add sketch "Sketch8" along normal blind 72 contours L0 L1 L2 L3 L4 L5 L6 bodies 1
sketch "Sketch9" plane through (-4.2795, 0, 33.3803) normal (0.127164, 0, -0.991882) x (0, 1, 0)
  line L0 (66, 152.3336) -> (72, 152.3336)
  line L1 (72, 152.3336) -> (72, 224.3336)
  line L2 (72, 224.3336) -> (66, 224.3336)
  line L3 (66, 224.3336) -> (66, 152.3336)
  line L4 (72, 224.3336) -> (66, 224.3336)
  line L5 (66, 224.3336) -> (66, 219.3336)
  line L6 (66, 219.3336) -> (72, 219.3336)
  line L7 (72, 219.3336) -> (72, 224.3336)
  dimension "d36" = 5
  constraint horizontal L4
  constraint vertical L5
  constraint horizontal L6
  constraint vertical L7
  constraint coincident L3 L5.end
  constraint coincident L1.end L2.start
  measures "d36" distance of L1.end L6.end
extrude "Extrude10" add sketch "Sketch9" along normal blind 40 contours L1 L2 L3 L4 L5 L6 L7 bodies 1
sketch "Sketch10" plane through (0.807, 0, -6.295) normal (0.127164, 0, -0.991882) x (0, 1, 0)
  line L0 (72, 219.3336) -> (72, 224.3336)
  line L1 (72, 224.3336) -> (66, 224.3336)
  line L2 (66, 224.3336) -> (66, 219.3336)
  line L3 (66, 219.3336) -> (72, 219.3336)
  line L4 (66, 219.3336) -> (72.721, 219.3336)
  line L5 (66, 214.8336) -> (66, 219.3336)
  line L6 (72, 219.3336) -> (66, 219.3336)
  line L7 (66, 219.3336) -> (66, 214.8336)
  line L8 (66, 214.8336) -> (72, 214.8336)
  line L9 (72, 214.8336) -> (72, 219.3336)
  line L10 (66, 214.8336) -> (72, 214.8336)
  line L11 (72, 214.8336) -> (72, 209.8336)
  line L12 (72, 209.8336) -> (66, 209.8336)
  line L13 (66, 209.8336) -> (66, 214.8336)
  dimension "d40" = 6
  dimension "d41" = 4.5
  dimension "d56" = 5
  constraint horizontal L4
  constraint vertical L5
  constraint coincident L2.end L3.start
  constraint horizontal L6
  constraint vertical L7
  constraint horizontal L8
  constraint vertical L9
  constraint coincident L0.start L3.end
  constraint horizontal L10
  constraint vertical L11
  constraint horizontal L12
  constraint vertical L13
  measures "d40" distance of L0.start L2.end
  measures "d41" distance of L0.start L8.end
  measures "d56" distance of L5.start L12.end
extrude "Extrude11" add sketch "Sketch10" against normal blind 5 contours L3 L4 L5 L6 L7 L8 L9 L10 bodies 1
extrude "Extrude13" add sketch "Sketch3" along normal blind 6 contours L0 L2 L7 L9 L10 L11 L12 bodies 1
sketch "Sketch11" plane through (-0.6856, 0, 5.348) normal (0.127164, 0, -0.991882) x (0, 1, 0)
  line L0 (66, 114.3824) -> (72, 114.3824)
  line L1 (72, 114.3824) -> (72, 152.3336)
  line L2 (72, 152.3336) -> (66, 152.3336)
  line L3 (66, 152.3336) -> (66, 114.3824)
  line L4 (72, 152.3336) -> (65.9909, 152.3336)
  line L5 (65.9909, 152.3336) -> (65.9909, 147.3336)
  line L6 (65.9909, 147.3336) -> (72, 147.3336)
  line L7 (72, 147.3336) -> (72, 152.3336)
  dimension "d49" = 5
  constraint horizontal L4
  constraint vertical L5
  constraint horizontal L6
  constraint vertical L7
  constraint coincident L1.end L2.start
  measures "d49" distance of L1.end L6.end
extrude "Extrude14" add sketch "Sketch11" along normal blind 4 contours L1 L2 L3 L4 L6 L7 bodies 1
fillet "Fillet4" radius 1 2 edges at (113.5311, 69, 13.9421) (108.5717, 69, 13.3062) on bodies 1
fillet "Fillet5" radius 1 2 edges at (145.9605, 69, 20.116) (150.9199, 69, 20.7519) on bodies 1
extrude "Extrude15" add sketch "Sketch10" against normal blind 11 separate body contours L8 L10 L11 L12 L13 makes body 2
fillet "Fillet6" radius 2 4 edges at (223.3194, 69, 22.2322) (212.4977, 69, 31.9349) (207.5383, 69, 31.2991) (208.9371, 69, 20.3884) on bodies 1 2
sketch "Sketch12" plane through (0, 66, 0) normal (0, -1, 0) x (1, 0, 0)
  arc A0 (221.3356, 21.9779) -> (223.0651, 24.216) centre (221.0813, 23.9617) ccw
  line L0 (223.0651, 24.216) -> (217.597, 66.8669)
  line L1 (217.597, 66.8669) -> (141.2221, 57.0753)
  line L2 (141.2221, 57.0753) -> (145.037, 27.3188)
  line L3 (145.037, 27.3188) -> (135.6529, 26.1157)
  line L4 (135.6529, 26.1157) -> (130, 28)
  line L5 (130, 28) -> (87, 28)
  line L6 (87, 28) -> (87, 17)
  line L7 (87, 17) -> (65, 17)
  line L8 (65, 17) -> (65, 6)
  line L9 (65, 6) -> (70, 6)
  line L10 (70, 6) -> (70, 12)
  line L11 (70, 12) -> (92, 12)
  line L12 (92, 12) -> (92, 23)
  line L13 (92, 23) -> (98, 23)
  line L14 (98, 23) -> (98, 18)
  line L15 (98, 18) -> (107.8087, 19.2575)
  line L16 (107.8087, 19.2575) -> (108.4445, 14.2981)
  arc A1 (108.4445, 14.2981) -> (109.5636, 13.4334) centre (109.4364, 14.4253) ccw
  line L17 (109.5636, 13.4334) -> (112.5392, 13.8149)
  arc A2 (112.5392, 13.8149) -> (113.4039, 14.9339) centre (112.4121, 14.8068) ccw
  line L18 (113.4039, 14.9339) -> (112.7681, 19.8933)
  line L19 (112.7681, 19.8933) -> (145.4518, 24.0836)
  line L20 (145.4518, 24.0836) -> (145.8333, 21.1079)
  arc A3 (145.8333, 21.1079) -> (146.9524, 20.2432) centre (146.8252, 21.2351) ccw
  line L21 (146.9524, 20.2432) -> (149.928, 20.6247)
  arc A4 (149.928, 20.6247) -> (150.7927, 21.7437) centre (149.8008, 21.6166) ccw
  line L22 (150.7927, 21.7437) -> (146.8173, 52.7517)
  line L23 (146.8173, 52.7517) -> (213.2734, 61.2717)
  line L24 (213.2734, 61.2717) -> (217.7242, 26.5558)
  line L25 (217.7242, 26.5558) -> (213.2607, 25.9836)
  line L26 (213.2607, 25.9836) -> (213.8965, 21.0242)
  line L27 (213.8965, 21.0242) -> (221.3356, 21.9779)
  line L28 (98, 23) -> (98.6307, 18.0809)
  constraint coincident L13.end L14.start
  constraint coincident L15 L28.end
  constraint perpendicular L15 L28
extrude "Extrude16" cut sketch "Sketch12" against normal blind 8 contours L14 L15 L28 bodies 1
fillet "Fillet7" radius 2 2 edges at (87, 69, 28) (65, 69, 17) on bodies 1
fillet "Fillet8" radius 2 2 edges at (141.2221, 69, 57.0753) (217.597, 69, 66.8669) on bodies 1
fillet "Fillet8" radius 2.5 2 edges at (146.8173, 69, 52.7517) (213.2734, 69, 61.2717) on bodies 1
sketch "Sketch13" plane through (0, 66, 0) normal (0, -1, 0) x (1, 0, 0)
  arc A0 (217.8513, 64.8832) -> (215.6132, 66.6126) centre (215.8676, 64.6288) ccw
  line L0 (215.6132, 66.6126) -> (143.2059, 57.3296)
  arc A1 (143.2059, 57.3296) -> (141.4764, 55.0915) centre (143.4602, 55.3458) ccw
  line L1 (141.4764, 55.0915) -> (145.037, 27.3188)
  line L2 (145.037, 27.3188) -> (135.6529, 26.1157)
  line L3 (135.6529, 26.1157) -> (130, 28)
  line L4 (130, 28) -> (89, 28)
  arc A2 (89, 28) -> (87, 26) centre (89, 26) ccw
  line L5 (87, 26) -> (87, 17)
  line L6 (87, 17) -> (67, 17)
  arc A3 (67, 17) -> (65, 15) centre (67, 15) ccw
  line L7 (65, 15) -> (65, 6)
  line L8 (65, 6) -> (70, 6)
  line L9 (70, 6) -> (70, 12)
  line L10 (70, 12) -> (92, 12)
  line L11 (92, 12) -> (92, 23)
  line L12 (92, 23) -> (98, 23)
  line L13 (98, 23) -> (98.6307, 18.0809)
  line L14 (98.6307, 18.0809) -> (107.8087, 19.2575)
  line L15 (107.8087, 19.2575) -> (108.4445, 14.2981)
  arc A4 (108.4445, 14.2981) -> (109.5636, 13.4334) centre (109.4364, 14.4253) ccw
  line L16 (109.5636, 13.4334) -> (112.5392, 13.8149)
  arc A5 (112.5392, 13.8149) -> (113.4039, 14.9339) centre (112.4121, 14.8068) ccw
  line L17 (113.4039, 14.9339) -> (112.7681, 19.8933)
  line L18 (112.7681, 19.8933) -> (145.4518, 24.0836)
  line L19 (145.4518, 24.0836) -> (145.8333, 21.1079)
  arc A6 (145.8333, 21.1079) -> (146.9524, 20.2432) centre (146.8252, 21.2351) ccw
  line L20 (146.9524, 20.2432) -> (149.928, 20.6247)
  arc A7 (149.928, 20.6247) -> (150.7927, 21.7437) centre (149.8008, 21.6166) ccw
  line L21 (150.7927, 21.7437) -> (147.1353, 50.272)
  arc A8 (149.2971, 53.0696) -> (147.1353, 50.272) centre (149.615, 50.5899) ccw
  line L22 (149.2971, 53.0696) -> (210.7937, 60.9538)
  arc A9 (213.5913, 58.792) -> (210.7937, 60.9538) centre (211.1116, 58.4741) ccw
  line L23 (213.5913, 58.792) -> (217.7242, 26.5558)
  line L24 (217.7242, 26.5558) -> (213.2607, 25.9836)
  line L25 (213.2607, 25.9836) -> (213.8965, 21.0242)
  line L26 (213.8965, 21.0242) -> (221.3356, 21.9779)
  arc A10 (221.3356, 21.9779) -> (223.0651, 24.216) centre (221.0813, 23.9617) ccw
  line L27 (223.0651, 24.216) -> (217.8513, 64.8832)
  line L28 (180.0454, 57.0117) -> (180.6812, 52.0523)
  line L29 (180.6812, 52.0523) -> (213.9092, 56.3123)
  line L30 (180.6812, 52.0523) -> (147.4532, 47.7923)
  dimension "d69" = 5
  constraint midpoint L22 L28.start
  constraint perpendicular L22 L28
  constraint coincident L23 L29.end
  constraint perpendicular L23 L29
  constraint coincident L21 L30.end
  constraint perpendicular L21 L30
  measures "d69" distance of L28.start L28.end
extrude "Extrude17" add sketch "Sketch13" against normal blind 6 contours L22 A9 L23 L28 L29 | L21 A8 L22 L28 L30 bodies 1
sketch "Sketch14" plane through (0, 66, 0) normal (0, -1, 0) x (1, 0, 0)
  arc A0 (217.8513, 64.8832) -> (215.6132, 66.6126) centre (215.8676, 64.6288) ccw
  line L0 (215.6132, 66.6126) -> (143.2059, 57.3296)
  arc A1 (143.2059, 57.3296) -> (141.4764, 55.0915) centre (143.4602, 55.3458) ccw
  line L1 (141.4764, 55.0915) -> (145.037, 27.3188)
  line L2 (145.037, 27.3188) -> (135.6529, 26.1157)
  line L3 (135.6529, 26.1157) -> (130, 28)
  line L4 (130, 28) -> (89, 28)
  arc A2 (89, 28) -> (87, 26) centre (89, 26) ccw
  line L5 (87, 26) -> (87, 17)
  line L6 (87, 17) -> (67, 17)
  arc A3 (67, 17) -> (65, 15) centre (67, 15) ccw
  line L7 (65, 15) -> (65, 6)
  line L8 (65, 6) -> (70, 6)
  line L9 (70, 6) -> (70, 12)
  line L10 (70, 12) -> (92, 12)
  line L11 (92, 12) -> (92, 23)
  line L12 (92, 23) -> (98, 23)
  line L13 (98, 23) -> (98.6307, 18.0809)
  line L14 (98.6307, 18.0809) -> (107.8087, 19.2575)
  line L15 (107.8087, 19.2575) -> (108.4445, 14.2981)
  arc A4 (108.4445, 14.2981) -> (109.5636, 13.4334) centre (109.4364, 14.4253) ccw
  line L16 (109.5636, 13.4334) -> (112.5392, 13.8149)
  arc A5 (112.5392, 13.8149) -> (113.4039, 14.9339) centre (112.4121, 14.8068) ccw
  line L17 (113.4039, 14.9339) -> (112.7681, 19.8933)
  line L18 (112.7681, 19.8933) -> (145.4518, 24.0836)
  line L19 (145.4518, 24.0836) -> (145.8333, 21.1079)
  arc A6 (145.8333, 21.1079) -> (146.9524, 20.2432) centre (146.8252, 21.2351) ccw
  line L20 (146.9524, 20.2432) -> (149.928, 20.6247)
  arc A7 (149.928, 20.6247) -> (150.7927, 21.7437) centre (149.8008, 21.6166) ccw
  line L21 (150.7927, 21.7437) -> (147.4532, 47.7923)
  line L22 (147.4532, 47.7923) -> (213.9092, 56.3123)
  line L23 (213.9092, 56.3123) -> (217.7242, 26.5558)
  line L24 (217.7242, 26.5558) -> (213.2607, 25.9836)
  line L25 (213.2607, 25.9836) -> (213.8965, 21.0242)
  line L26 (213.8965, 21.0242) -> (221.3356, 21.9779)
  arc A8 (221.3356, 21.9779) -> (223.0651, 24.216) centre (221.0813, 23.9617) ccw
  line L27 (223.0651, 24.216) -> (217.8513, 64.8832)
  line L28 (213.9092, 56.3123) -> (213.2734, 61.2717) construction
  line L29 (213.2734, 61.2717) -> (141.8579, 52.1159) construction
  line L30 (141.8579, 52.1159) -> (218.2328, 61.9075)
  dimension "d72" = 5
  constraint coincident L22.end L23.start
  constraint perpendicular L22 L28
  constraint coincident L1 L29.end
  constraint perpendicular L1 L29
  constraint coincident L27 L30.end
  constraint perpendicular L27 L30
  measures "d72" distance of L22.end L28.end
extrude "Extrude18" cut sketch "Sketch14" against normal blind 10 contours A0 L0 A1 L1 L27 L30 bodies 1
fillet "Fillet9" radius 2 2 edges at (218.2328, 69, 61.9075) (141.8579, 69, 52.1159) on bodies 1
fillet "Fillet10" radius 1 2 edges at (213.9092, 69, 56.3123) (147.4532, 69, 47.7923) on bodies 1
combine "Combine1" operation add target body 2 tool bodies 1
sketch "Sketch15" plane through (0, 66, 0) normal (0, -1, 0) x (1, 0, 0)
  arc A0 (208.6828, 22.3721) -> (210.9209, 20.6427) centre (210.6666, 22.6265) ccw
  line L0 (210.9209, 20.6427) -> (221.3356, 21.9779)
  arc A1 (221.3356, 21.9779) -> (223.0651, 24.216) centre (221.0813, 23.9617) ccw
  line L1 (223.0651, 24.216) -> (218.4872, 59.9237)
  arc A2 (218.4872, 59.9237) -> (216.2491, 61.6532) centre (216.5034, 59.6694) ccw
  line L2 (216.2491, 61.6532) -> (143.8417, 52.3702)
  arc A3 (143.8417, 52.3702) -> (142.1123, 50.1321) centre (144.096, 50.3864) ccw
  line L3 (142.1123, 50.1321) -> (145.037, 27.3188)
  line L4 (145.037, 27.3188) -> (135.6529, 26.1157)
  line L5 (135.6529, 26.1157) -> (130, 28)
  line L6 (130, 28) -> (89, 28)
  arc A4 (89, 28) -> (87, 26) centre (89, 26) ccw
  line L7 (87, 26) -> (87, 17)
  line L8 (87, 17) -> (67, 17)
  arc A5 (67, 17) -> (65, 15) centre (67, 15) ccw
  line L9 (65, 15) -> (65, 6)
  line L10 (65, 6) -> (70, 6)
  line L11 (70, 6) -> (70, 12)
  line L12 (70, 12) -> (92, 12)
  line L13 (92, 12) -> (92, 23)
  line L14 (92, 23) -> (98, 23)
  line L15 (98, 23) -> (98.6307, 18.0809)
  line L16 (98.6307, 18.0809) -> (107.8087, 19.2575)
  line L17 (107.8087, 19.2575) -> (108.4445, 14.2981)
  arc A6 (108.4445, 14.2981) -> (109.5636, 13.4334) centre (109.4364, 14.4253) ccw
  line L18 (109.5636, 13.4334) -> (112.5392, 13.8149)
  arc A7 (112.5392, 13.8149) -> (113.4039, 14.9339) centre (112.4121, 14.8068) ccw
  line L19 (113.4039, 14.9339) -> (112.7681, 19.8933)
  line L20 (112.7681, 19.8933) -> (145.4518, 24.0836)
  line L21 (145.4518, 24.0836) -> (145.8333, 21.1079)
  arc A8 (145.8333, 21.1079) -> (146.9524, 20.2432) centre (146.8252, 21.2351) ccw
  line L22 (146.9524, 20.2432) -> (149.928, 20.6247)
  arc A9 (149.928, 20.6247) -> (150.7927, 21.7437) centre (149.8008, 21.6166) ccw
  line L23 (150.7927, 21.7437) -> (147.5803, 46.8004)
  arc A10 (148.4451, 47.9194) -> (147.5803, 46.8004) centre (148.5722, 46.9276) ccw
  line L24 (148.4451, 47.9194) -> (212.9174, 56.1851)
  arc A11 (214.0364, 55.3204) -> (212.9174, 56.1851) centre (213.0445, 55.1932) ccw
  line L25 (214.0364, 55.3204) -> (217.7242, 26.5558)
  line L26 (217.7242, 26.5558) -> (213.2607, 25.9836)
  line L27 (213.2607, 25.9836) -> (212.752, 29.9511)
  arc A12 (212.752, 29.9511) -> (210.514, 31.6806) centre (210.7683, 29.6968) ccw
  line L28 (210.514, 31.6806) -> (209.5221, 31.5534)
  arc A13 (209.5221, 31.5534) -> (207.7926, 29.3153) centre (209.7764, 29.5696) ccw
  line L29 (207.7926, 29.3153) -> (208.6828, 22.3721)

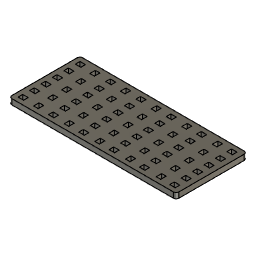
design "Component Carrier"
Autodesk Fusion 360 part; units mm, degrees